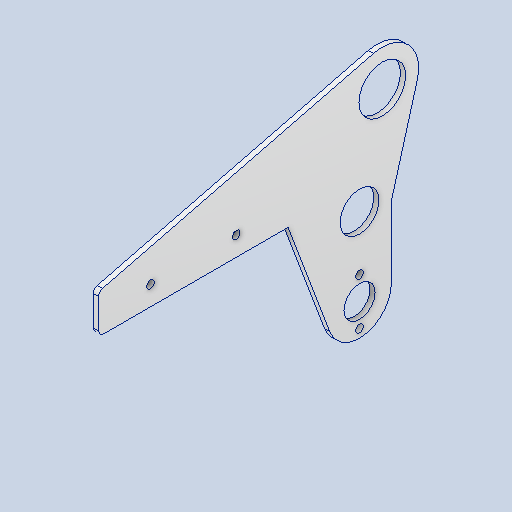
# Autodesk Inventor part: RZvector-arm-rotate-v1-Plate-MM5-F-R
Saved by Autodesk Inventor 2024 (Build 280153000, 153)
## iProperties
Created: 2024-03-10
Part Number: RZvector-arm-rotate-v1-Plate-MM5-F-R
Material: アルミニウム 6061
Document SubType Name: Modeling
Designer: haruy
Density: 2.7 g/cm^3
Appearance: アルミニウム - フラット
Mass: 9.04662 g
Surface Area: 101.451 cm^2
Volume: 9.04662 cm^3
Author: haruy
Autodesk Inventor part; units mm, degrees
ref_plane "YZ Plane" through (0, 0, 0) normal (1, 0, 0) x (0, 1, 0)
ref_plane "XZ Plane" through (0, 0, 0) normal (0, 1, 0) x (-1, 0, 0)
ref_plane "XY Plane" through (0, 0, 0) normal (0, 0, 1) x (1, 0, 0)
derived "RZvector-arm-rotate-v1-Sketch-Base.ipt"
sketch "横から" plane through (0, 0, 0) normal (1, 0, 0) x (0, 1, 0)
  line L0 (0, 0) -> (0, -30.2937)
  line L1 (542.7807, -196.25) -> (0, -196.25)
  line L2 (628, -186.25) -> (24, -186.25)
  line L3 (24, -186.25) -> (24, -206.25)
  line L4 (24, -206.25) -> (628, -206.25)
  line L5 (628, -206.25) -> (628, -186.25)
  line L6 (138, -159.75) -> (123, -159.75)
  line L7 (123, -159.75) -> (123, -174.75)
  line L8 (123, -174.75) -> (138, -174.75)
  line L9 (138, -174.75) -> (138, -159.75)
  line L10 (0, 0) -> (0, -196.25)
  line L11 (138, -217.75) -> (123, -217.75)
  line L12 (123, -217.75) -> (123, -232.75)
  line L13 (123, -232.75) -> (138, -232.75)
  line L14 (138, -232.75) -> (138, -217.75)
  line L15 (0, 0) -> (0, -415.25)
  line L16 (54, -415.25) -> (34, -415.25)
  line L17 (34, -415.25) -> (34, -395.25)
  line L18 (34, -395.25) -> (54, -395.25)
  line L19 (54, -395.25) -> (54, -415.25)
  line L20 (134, -345.25) -> (64, -345.25)
  line L21 (64, -345.25) -> (64, -395.25)
  line L22 (64, -395.25) -> (134, -395.25)
  line L23 (134, -395.25) -> (134, -345.25)
  line L24 (136, -310.25) -> (134, -310.25)
  line L25 (134, -310.25) -> (134, -405.25)
  line L26 (134, -405.25) -> (136, -405.25)
  line L27 (136, -405.25) -> (136, -310.25)
  line L28 (136, -310.25) -> (146, -310.25)
  line L29 (146, -310.25) -> (146, -320.25)
  line L30 (146, -320.25) -> (136, -320.25)
  line L31 (136, -320.25) -> (136, -310.25)
  line L32 (146, -320.25) -> (54, -320.25)
  line L33 (54, -320.25) -> (54, -330.25)
  line L34 (54, -330.25) -> (146, -330.25)
  line L35 (146, -330.25) -> (146, -320.25)
  line L36 (0, -269) -> (385.3867, -269)
  line L37 (144, 54.75) -> (46, 54.75)
  line L38 (46, 54.75) -> (46, -139.45)
  line L39 (46, -139.45) -> (144, -139.45)
  line L40 (144, -139.45) -> (144, 54.75)
  circle A0 centre (95, 2.25) radius 95
  line L41 (176, -92.75) -> (156, -92.75)
  line L42 (156, -92.75) -> (156, -290.75)
  line L43 (156, -290.75) -> (176, -290.75)
  line L44 (176, -290.75) -> (176, -92.75)
  circle A1 centre (166, -269) radius 6
  circle A2 centre (166, -269) radius 22.5
  circle A3 centre (129.5351, -260.25) radius 15
  circle A4 centre (129.5351, -260.25) radius 6
  line L45 (138, -159.75) -> (153, -159.75)
  line L46 (153, -159.75) -> (153, -232.75)
  line L47 (153, -232.75) -> (138, -232.75)
  line L48 (138, -232.75) -> (138, -159.75)
  line L49 (123, -174.75) -> (153, -174.75)
  line L50 (153, -174.75) -> (153, -184.75)
  line L51 (153, -184.75) -> (123, -184.75)
  line L52 (123, -184.75) -> (123, -174.75)
  line L53 (123, -217.75) -> (153, -217.75)
  line L54 (153, -217.75) -> (153, -207.75)
  line L55 (153, -207.75) -> (123, -207.75)
  line L56 (123, -207.75) -> (123, -217.75)
  circle A5 centre (129.5351, -260.25) radius 18.75
  circle A6 centre (99.5351, -260.25) radius 15
  circle A7 centre (145.5, -179.75) radius 1.5
  circle A8 centre (145.5, -212.75) radius 1.5
  circle A9 centre (166, -269) radius 14
  circle A10 centre (166, -269) radius 9
  circle A11 centre (129.5351, -260.25) radius 7.5
  circle A12 centre (99.5351, -260.25) radius 6
  circle A13 centre (99.5351, -260.25) radius 12.25
  circle A14 centre (99.5351, -260.25) radius 9
  circle A15 centre (108.5351, -260.25) radius 1.5
  circle A16 centre (90.5351, -260.25) radius 1.5
  line L57 (153, -159.75) -> (179.5784, -265.5902)
  circle A17 centre (129.5351, -260.25) radius 12.5
  line L58 (162.1914, -282.472) -> (126.1346, -272.2786)
  line L59 (129.431, -272.7496) -> (99.433, -272.4996)
  line L60 (138, -232.75) -> (95.2356, -248.7793)
  line L61 (136, -330.25) -> (146, -330.25)
  line L62 (146, -330.25) -> (146, -340.25)
  line L63 (146, -340.25) -> (136, -340.25)
  line L64 (136, -340.25) -> (136, -330.25)
  line L65 (54, -405.25) -> (56, -405.25)
  line L66 (56, -405.25) -> (56, -345.2512)
  line L67 (56, -345.2512) -> (54, -345.2512)
  line L68 (54, -345.2512) -> (54, -405.25)
  line L69 (56, -320.25) -> (64.683, -320.25)
  line L70 (54, -310.25) -> (64, -310.25)
  line L71 (64, -310.25) -> (64, -320.25)
  line L72 (64, -320.25) -> (54, -320.25)
  line L73 (54, -320.25) -> (54, -310.25)
  line L74 (54, -310.25) -> (44, -310.25)
  line L75 (44, -310.25) -> (44, -340.25)
  line L76 (44, -340.25) -> (54, -340.25)
  line L77 (54, -340.25) -> (54, -310.25)
  line L78 (34, -415.25) -> (54, -415.25)
  line L79 (54, -415.25) -> (54, -139.45)
  line L80 (54, -139.45) -> (34, -139.45)
  line L81 (34, -139.45) -> (34, -415.25)
  line L82 (628, -186.25) -> (659.5, -186.25)
  line L83 (659.5, -186.25) -> (659.5, -206.25)
  line L84 (659.5, -206.25) -> (628, -206.25)
  line L85 (628, -206.25) -> (628, -186.25)
  line L86 (54, -375.25) -> (34, -375.25)
  circle A18 centre (129.5351, -260.25) radius 12.5
  circle A19 centre (643.75, -167.5) radius 15.75
  line L87 (659.5, -186.25) -> (659.5, -167.5)
  line L88 (628, -186.25) -> (628, -167.5)
  line L89 (150.5, -293.5212) -> (150.5, -446.3995)
  line L90 (34, -395.25) -> (477, -395.25)
  line L91 (477, -395.25) -> (477, -375.25)
  line L92 (477, -375.25) -> (34, -375.25)
  line L93 (34, -375.25) -> (34, -395.25)
  line L94 (184, -375.25) -> (194, -375.25)
  line L95 (194, -375.25) -> (194, -365.25)
  line L96 (194, -365.25) -> (184, -365.25)
  line L97 (184, -365.25) -> (184, -375.25)
  line L98 (230, -365.25) -> (194, -365.25)
  line L99 (194, -365.25) -> (194, -399.25)
  line L100 (194, -399.25) -> (230, -399.25)
  line L101 (230, -399.25) -> (230, -365.25)
  line L102 (212, -365.25) -> (212, -399.25)
  line L103 (194, -365.25) -> (204, -365.25)
  line L104 (204, -365.25) -> (204, -395.25)
  line L105 (204, -395.25) -> (194, -395.25)
  line L106 (194, -395.25) -> (194, -365.25)
  line L107 (423, -49.3886) -> (335, -49.3886)
  line L108 (335, -49.3886) -> (335, -349.3886)
  line L109 (335, -349.3886) -> (423, -349.3886)
  line L110 (423, -349.3886) -> (423, -49.3886)
  line L111 (394, -349.3886) -> (364, -349.3886)
  line L112 (364, -349.3886) -> (364, -369.3886)
  line L113 (364, -369.3886) -> (394, -369.3886)
  line L114 (394, -369.3886) -> (394, -349.3886)
  line L115 (359, -365.25) -> (349, -365.25)
  line L116 (349, -365.25) -> (349, -375.25)
  line L117 (349, -375.25) -> (359, -375.25)
  line L118 (359, -375.25) -> (359, -365.25)
  line L119 (379, -349.3886) -> (379, -369.3886)
  line L120 (347, -375.25) -> (357, -375.25)
  line L121 (521, -49.3886) -> (433, -49.3886)
  line L122 (433, -49.3886) -> (433, -349.3886)
  line L123 (433, -349.3886) -> (521, -349.3886)
  line L124 (521, -349.3886) -> (521, -49.3886)
  line L125 (457, -375.25) -> (447, -375.25)
  line L126 (447, -375.25) -> (447, -365.25)
  line L127 (447, -365.25) -> (457, -365.25)
  line L128 (457, -365.25) -> (457, -375.25)
  line L129 (643.186, -209.9292) -> (479.1599, -376.8167)
  line L130 (479.1599, -376.8167) -> (493.4238, -390.836)
  line L131 (493.4238, -390.836) -> (657.4499, -223.9485)
  line L132 (657.4499, -223.9485) -> (643.186, -209.9292)
  line L133 (457, -375.25) -> (457, -395.25)
  line L134 (493.1793, -362.5528) -> (507.4432, -376.5721)
  line L135 (629.1667, -224.1931) -> (643.4306, -238.2124)
  line L136 (230, -375.25) -> (220, -375.25)
  line L137 (220, -375.25) -> (220, -365.25)
  line L138 (220, -365.25) -> (230, -365.25)
  line L139 (230, -365.25) -> (230, -375.25)
  line L140 (230, -365.25) -> (65, -365.25)
  line L141 (65, -365.25) -> (65, -360.25)
  line L142 (65, -360.25) -> (230, -360.25)
  line L143 (230, -360.25) -> (230, -365.25)
  line L144 (220, -309.25) -> (65, -309.25)
  line L145 (65, -309.25) -> (65, -313.25)
  line L146 (65, -313.25) -> (220, -313.25)
  line L147 (220, -313.25) -> (220, -309.25)
  line L148 (65, -365.25) -> (70, -365.25)
  line L149 (70, -365.25) -> (70, -309.25)
  line L150 (70, -309.25) -> (65, -309.25)
  line L151 (65, -309.25) -> (65, -365.25)
  line L152 (239, -375.25) -> (239, -395.25)
  line L153 (130, -371.7504) -> (108.5351, -371.7504)
  line L154 (108.5351, -371.7504) -> (108.5351, -456.25)
  line L155 (108.5351, -456.25) -> (130, -456.25)
  line L156 (130, -456.25) -> (130, -371.7504)
  circle A20 centre (175, -269) radius 6
  line L157 (302.5611, -391.0338) -> (151.9649, -262.485)
  line L158 (151.9649, -262.485) -> (164.9496, -247.2732)
  line L159 (164.9496, -247.2732) -> (315.5458, -375.822)
  line L160 (315.5458, -375.822) -> (302.5611, -391.0338)
  circle A21 centre (427.4049, -391.1037) radius 95
  line L161 (900, 0) -> (900, -1750.1016)
  line L162 (525, -456.25) -> (0, -456.25)
  line L163 (0, -456.25) -> (0, -706.25)
  line L164 (0, -706.25) -> (525, -706.25)
  line L165 (525, -706.25) -> (525, -456.25)
  line L166 (286.9304, -332.3317) -> (437.1463, -460.5559)
  line L167 (437.1463, -460.5559) -> (497.5252, -389.8213)
  line L168 (497.5252, -389.8213) -> (347.3093, -261.5971)
  line L169 (347.3093, -261.5971) -> (286.9304, -332.3317)
  line L170 (659.5, -186.25) -> (668.5, -186.25)
  line L171 (668.5, -186.25) -> (668.5, -206.25)
  line L172 (668.5, -206.25) -> (659.5, -206.25)
  line L173 (659.5, -206.25) -> (659.5, -186.25)
  line L174 (224, -174.75) -> (194, -174.75)
  line L175 (194, -174.75) -> (194, -217.75)
  line L176 (194, -217.75) -> (224, -217.75)
  line L177 (224, -217.75) -> (224, -174.75)
  line L178 (605, -186.25) -> (605, -206.25)
  line L179 (242.3, -171.25) -> (226.4, -171.25)
  line L180 (226.4, -171.25) -> (226.4, -199.05)
  line L181 (226.4, -199.05) -> (242.3, -199.05)
  line L182 (242.3, -199.05) -> (242.3, -171.25)
  circle A22 centre (239.5, -196.25) radius 1.7
  circle A23 centre (229.2, -174.05) radius 1.7
  circle A24 centre (247.5, -196.25) radius 1.7
  line L183 (252.5, -186.25) -> (252.5, -206.25)
  line L184 (550.2984, 177.2044) -> (550.2984, -1079.3945)
  line L185 (477, -375.25) -> (590, -375.25)
  line L186 (590, -375.25) -> (590, -395.25)
  line L187 (590, -395.25) -> (477, -395.25)
  line L188 (477, -395.25) -> (477, -375.25)
  line L189 (590, -395.25) -> (578, -395.25)
  line L190 (578, -395.25) -> (578, -407.25)
  line L191 (578, -407.25) -> (590, -407.25)
  line L192 (590, -407.25) -> (590, -395.25)
  line L193 (239, -375.25) -> (229, -375.25)
  line L194 (229, -375.25) -> (229, -365.25)
  line L195 (229, -365.25) -> (239, -365.25)
  line L196 (239, -365.25) -> (239, -375.25)
  line L197 (245.8, -370.25) -> (224.6774, -352.1759)
  line L198 (224.6774, -352.1759) -> (236.9001, -337.8915)
  line L199 (236.9001, -337.8915) -> (258.0228, -355.9656)
  line L200 (258.0228, -355.9656) -> (245.8, -370.25)
  circle A25 centre (247.3784, -364.0987) radius 1.7
  circle A26 centre (237.2072, -341.8394) radius 1.7
  line L201 (239, -365.25) -> (249, -365.25)
  line L202 (249, -365.25) -> (249, -375.25)
  line L203 (249, -375.25) -> (239, -375.25)
  line L204 (239, -375.25) -> (239, -365.25)
  line L205 (249, -365.25) -> (224.6774, -365.25)
  line L206 (224.6774, -365.25) -> (224.6774, -355.25)
  line L207 (224.6774, -355.25) -> (249, -355.25)
  line L208 (249, -355.25) -> (249, -365.25)
  line L209 (224.6774, -365.25) -> (230, -365.25)
  line L210 (230, -365.25) -> (230, -375.25)
  line L211 (230, -375.25) -> (224.6774, -375.25)
  line L212 (224.6774, -375.25) -> (224.6774, -365.25)
  line L213 (224.6774, -352.1759) -> (224.6774, -355.25)
  line L214 (239, -368.75) -> (249, -368.75)
  line L215 (249, -368.75) -> (249, -371.75)
  line L216 (249, -371.75) -> (239, -371.75)
  line L217 (239, -371.75) -> (239, -368.75)
  line L218 (258.0228, -355.9656) -> (249, -375.25)
  line L219 (593.9382, -399.979) -> (576.2016, -378.5721)
  line L220 (576.2016, -378.5721) -> (590.6782, -366.5776)
  line L221 (590.6782, -366.5776) -> (608.4148, -387.9845)
  line L222 (608.4148, -387.9845) -> (593.9382, -399.979)
  circle A27 centre (596.5409, -394.1863) radius 1.7
  circle A28 centre (590.3086, -370.5201) radius 1.7
  line L223 (590, -407.25) -> (600, -407.25)
  line L224 (600, -407.25) -> (600, -397.25)
  line L225 (600, -397.25) -> (590, -397.25)
  line L226 (590, -397.25) -> (590, -407.25)
  line L227 (600, -397.25) -> (576.2016, -397.25)
  line L228 (576.2016, -397.25) -> (576.2016, -378.5721)
  line L229 (576.2016, -378.5721) -> (600, -378.5721)
  line L230 (600, -378.5721) -> (600, -397.25)
  line L231 (576.2016, -397.25) -> (578, -397.25)
  line L232 (578, -397.25) -> (578, -407.25)
  line L233 (578, -407.25) -> (576.2016, -407.25)
  line L234 (576.2016, -407.25) -> (576.2016, -397.25)
  line L235 (608.4148, -387.9845) -> (600, -407.25)
  line L236 (590, -375.25) -> (610, -375.25)
  line L237 (610, -375.25) -> (610, -395.25)
  line L238 (610, -395.25) -> (590, -395.25)
  line L239 (590, -395.25) -> (590, -375.25)
  line L240 (648.5, -186.25) -> (648.5, -206.25)
  line L241 (667.9052, -217.2444) -> (610, -371.75)
  line L242 (610, -371.75) -> (591.272, -364.7312)
  line L243 (591.272, -364.7312) -> (649.1773, -210.2256)
  line L244 (649.1773, -210.2256) -> (667.9052, -217.2444)
  line L245 (660.8864, -235.9723) -> (642.1585, -228.9535)
  line L246 (617.0188, -353.022) -> (598.2909, -346.0032)
  point P0 (166, -92.75)
  point P1 (98.012, -272.4049)
  point P2 (176, -259.202)
  point P3 (176, -251.3403)
  point P4 (176, -278.798)
  point P5 (156, -280.7217)
  point P6 (156, -171.6966)
  point P7 (127.7511, -272.7356)
  point P8 (156, -278.798)
  point P9 (156, -259.202)
  point P10 (101.6417, -269)
  point P11 (97.4286, -269)
  point P12 (394, -359.3886)
  point P13 (643.75, -206.25)
  point P14 (247.4615, -346.9286)
  dimension "d12" = 18
  dimension "d1" = 3
  dimension "d2" = 3
  dimension "d3" = 7.5
  dimension "d4" = 7.5
  dimension "d5" = 5
  dimension "d6" = 5
  dimension "d7" = 28
  dimension "d8" = 18
  dimension "d9" = 15
  dimension "d10" = 12
  dimension "d11" = 24.5
  dimension "d13" = 3
  dimension "d16" = 360
  dimension "d18" = 25
  measures "d1" diameter of A7
  measures "d2" diameter of A8
  measures "d3" distance from line of A7.centre L46
  measures "d4" distance from line of A8.centre L46
  measures "d5" distance from line of A7.centre L49
  measures "d6" distance from line of A8.centre L53
  measures "d7" diameter of A9
  measures "d8" diameter of A10
  measures "d9" diameter of A11
  measures "d10" diameter of A12
  measures "d11" diameter of A13
  measures "d13" diameter of A15
  measures "d18" diameter of A17
extrude "押し出し1" add sketch "横から" along normal blind 2 contours L159 L44 L57 | L57 A20 A9 L44 L159 | L57 A2 L42 L4 | L4 L42 L1 L57 | A9 A20 L44 L36 | L36 L44 A20 A9 | L57 A9 A20 | A9 L44 A20 | L44 L159 L158 L42 A2 L57 | L44 A9 L42 L158 L159 | L42 A2 A5 A6 L60 L47 L46 L4 | L4 L46 L1 L42 | L1 L42 L2 L57 | L44 A20 A10 L36 | L36 A10 A20 L44 | A20 L44 A9 | A9 L157 A10 A20 L44 | A9 L42 L36 A10 L157 | L42 L158 L157 A9 L36 A5 A2 | L44 A20 A10 L157 L42 A9 | L2 L42 L57 | L46 L55 L48 L4 | L4 L48 L1 L46 | L1 L46 L2 L42 | L58 L42 A9 | L42 A9 L157 L158 | A5 L36 A2 | A2 A3 A6 A5 | L42 L157 A9 | L2 L46 L57 L42 | L1 L48 L2 L46 | L46 L53 L48 L55 | A9 L36 L42 | L42 L58 A2 A5 L36 A9 | L36 L42 L157 A10 | A2 L36 A3 | A3 L36 A17 | A6 A5 A13 | A5 A13 L60 A6 | L42 L36 A9 L157 | L2 L48 L51 L46 | L46 L49 L9 L45 | L46 L47 L14 L53 | L58 A5 A2 | A2 A5 L58 A3 L36 | L36 A5 A2 | A3 L58 L59 A17 L36 | A13 A5 | A5 A13 L36 A14 A15 A16 | A3 L36 A5 A6 | L51 L48 L49 L46 | A17 L36 | L36 A17 | A5 A6 L36 A13 | A3 L59 A5 L36 | L36 A17 L58 L59 A3 | A5 L36 A6 | L59 A6 L36 A5 | L59 L58 A17 | A13 L36 A14 | L36 A6 L59 A13 | A14 L36 | L36 A14 A16 A15 picked at (107.9273, -270.341)
fillet "フィレット1" radius 2 2 edges at (1, 153, -159.75) (1, 138, -159.75)
